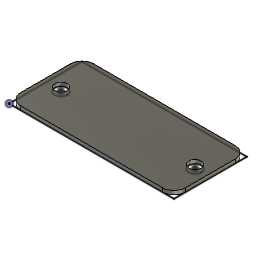
Famicom Box Coinbox Cover Small v1 (Autodesk Fusion 360 design; units mm, degrees)
Autodesk Fusion 360 part; units mm, degrees
sketch "Sketch1" plane through (0, 0, 0) normal (0, 0, 1) x (1, 0, 0)
  line L0 (0, 0) -> (43, 0)
  line L1 (43, 0) -> (43, 19)
  line L2 (43, 19) -> (0, 19)
  line L3 (0, 19) -> (0, 0)
  circle A0 centre (39, 9.5) radius 1.6
  circle A1 centre (4, 9.5) radius 1.6
  dimension "d1" = 43
  dimension "d2" = 19
  dimension "d3" = 3.2
  dimension "d4" = 3.2
  dimension "d5" = 4
  dimension "d6" = 4
  dimension "d17" = 9.5
  dimension "d18" = 9.5
  constraint horizontal L0
  constraint vertical L1
  constraint horizontal L2
  constraint vertical L3
  constraint coincident L0.start L3.end
  measures "d1" distance of L1.end L2.end
  measures "d2" distance of L0 L2
  measures "d3" diameter of A0
  measures "d4" diameter of A1
  measures "d5" distance of L3 A1.centre
  measures "d6" distance of L1 A0.centre
  measures "d17" distance of L2 A1.centre
  measures "d18" distance of L2 A0.centre
extrude "Extrude1" add sketch "Sketch1" along normal blind 1
fillet "Fillet1" radius 3 1 edges at (43, 19, 0.5)
fillet "Fillet1" radius 3 1 edges at (0, 19, 0.5)
fillet "Fillet1" radius 3 1 edges at (0, 0, 0.5)
fillet "Fillet1" radius 3 1 edges at (43, 0, 0.5)
